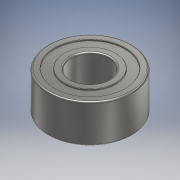
# Autodesk Inventor part: 685zz
Saved by Autodesk Inventor 2017 (Build 210142000, 142)
## iProperties
Created: 2016-06-20
Part Number: 685zz
Material: Stainless Steel
Document SubType Name: Modeling
Designer: hmigu
Density: 8 g/cm^3
Appearance: Semi-Polished
Author: hmigu
Autodesk Inventor part; units mm, degrees
ref_plane "YZ Plane" through (0, 0, 0) normal (1, 0, 0) x (0, 1, 0)
ref_plane "XZ Plane" through (0, 0, 0) normal (0, 1, 0) x (-1, 0, 0)
ref_plane "XY Plane" through (0, 0, 0) normal (0, 0, 1) x (1, 0, 0)
sketch "Sketch1" plane through (0, 0, 0) normal (0, 1, 0) x (-1, 0, 0)
  line L0 (0, -1.9986) -> (0, 1.9986)
  line L1 (5.5, -2.5) -> (4.6, -2.5)
  line L2 (4.6, 2.5) -> (5.5, 2.5)
  line L3 (5.5, 2.5) -> (5.5, -2.5)
  line L4 (4.6, -2.3327) -> (3.4, -2.3327)
  line L5 (3.4, 2.3327) -> (4.6, 2.3327)
  line L6 (3.4, -2.5) -> (2.5, -2.5)
  line L7 (2.5, -2.5) -> (2.5, 2.5)
  line L8 (2.5, 2.5) -> (3.4, 2.5)
  line L9 (3.4, 2.5) -> (3.4, 2.3327)
  line L10 (3.4, -2.3327) -> (3.4, -2.5)
  line L11 (4.6, -2.5) -> (4.6, -2.3327)
  line L12 (4.6, 2.3327) -> (4.6, 2.5)
  point P0 (0, 0)
  point P1 (0, 0)
  point P2 (2.5, 0)
  dimension "d0" = 5
  dimension "d1" = 11
  dimension "d2" = 5
  dimension "d4" = 1.2
  dimension "d9" = 0.1673
  constraints: 26 end point, 7 parallel, 4 collinear, 3 horizontal, 3 perpendicular, 2 midpoint, 2 point on line, 1 coincident, 1 horizontal alignment, 1 vertical
  measures "d0" diameter of L7 L0
  measures "d1" diameter of L3 L0
  measures "d2" distance of L2.end L1.start
  measures "d4" distance of L4.start L4.end
  measures "d9" distance of L1.end L4.start
revolve "Revolution1" add sketch "Sketch1" angle 360 about axis through (0, 0, -1.9986) along (0, 0, 1)
fillet "Fillet1" radius 0.2 4 edges at (5.5, 0, 2.5) (2.5, 0, 2.5) (5.5, 0, -2.5) (2.5, 0, -2.5)
fillet "Fillet2" radius 0.05 4 edges at (4.6, 0, 2.5) (3.4, 0, 2.5) (3.4, 0, -2.5) (4.6, 0, -2.5)
body "Solid1"
